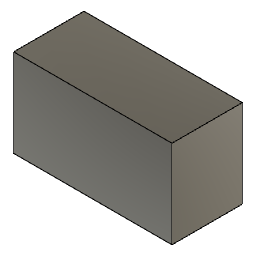
KonsoleTischSupports v2 (Autodesk Fusion 360 design; units mm, degrees)
Autodesk Fusion 360 part; units mm, degrees
note: some values were not read from the file. Chosen so that the rebuilt part matches the saved one: which face or edge a step refers to.
sketch "Main" plane through (0, 0, 0) normal (0, 0, 1) x (1, 0, 0)
  line L0 (90, 40) -> (-90, 40)
  line L1 (-90, 40) -> (-90, -40)
  line L2 (-90, -40) -> (90, -40)
  line L3 (90, -40) -> (90, 40)
  line L4 (90, 40) -> (-90, -40) construction
  line L5 (-90, 40) -> (90, -40) construction
  dimension "d7" = 80
  dimension "d8" = 180
  constraint horizontal L0
  constraint perpendicular L0 L1
  constraint parallel L0 L2
  constraint parallel L1 L3
  constraint coincident L4 origin
  constraint coincident L5 origin
  measures "d7" distance of L0.end L1.end
  measures "d8" distance of L0.start L0.end
extrude "Extrude1" add sketch "Main" along normal blind 100
shell "Shell1" thickness 3 removed faces 0 bodies 1
sketch "Sketch6" plane through (0, 0, 0) normal (0, 0, -1) x (1, 0, 0)
  line L0 (90, -40) -> (90, 40)
  line L1 (90, 40) -> (-90, 40)
  line L2 (-90, 40) -> (-90, -40)
  line L3 (-90, -40) -> (90, -40)
  circle A0 centre (0, 0) radius 25
  dimension "d25" = 50
  constraint coincident A0.centre origin
  measures "d25" diameter of A0
extrude "Extrude5" cut sketch "Sketch6" against normal blind 10 draft -30 contours A0
sketch "ThinnerSketch" plane through (0, 0, -10) normal (0, 0, -1) x (1, 0, 0)
  circle A0 centre (0, 0) radius 25
  line L0 (90, 40) -> (-90, 40)
  line L1 (-90, 40) -> (-90, -40)
  line L2 (-90, -40) -> (90, -40)
  line L3 (90, -40) -> (90, 40)
  line L4 (87, 37) -> (-87, 37)
  line L5 (-87, 37) -> (-87, -37)
  line L6 (-87, -37) -> (87, -37)
  line L7 (87, -37) -> (87, 37)
  line L8 (87, 37) -> (-87, -37) construction
  line L9 (-87, 37) -> (87, -37) construction
  dimension "d20" = 74
  dimension "d21" = 174
  constraint horizontal L4
  constraint perpendicular L4 L5
  constraint parallel L4 L6
  constraint parallel L5 L7
  constraint coincident L8 A0.centre
  constraint coincident L9 A0.centre
  constraint coincident A0.centre origin
  measures "d20" distance of L4.end L5.end
  measures "d21" distance of L4.start L4.end
extrude "Extrude4" [rolled back] along distance 10 taper angle 0
sketch "Sketch2" plane through (0, 0, 100) normal (0, 0, 1) x (-1, 0, 0)
  line L0 (-90, 40) -> (-90, -40)
  line L1 (-90, -40) -> (90, -40)
  line L2 (90, -40) -> (90, 40)
  line L3 (90, 40) -> (-90, 40)
equation "base_length = 18 cm"
equation "base_width = 8 cm"
equation "shell_thickness = 3 mm"
equation "base_thickness = 10 mm"
equation "hole_diameter = 5 cm"
equation "hole_taper_angle = -30 deg"
equation "d7 = base_width"
equation "d8 = base_length"
equation "d9 = base_height"
equation "base_height = 10 cm"
equation "d12 = shell_thickness"
equation "d20 = base_width - shell_thickness - shell_thickness"
equation "d21 = base_length - shell_thickness - shell_thickness"
equation "d22 = -base_thickness - shell_thickness"
equation "d25 = hole_diameter"
equation "d27 = hole_taper_angle"
named bodies: "MainBody"
